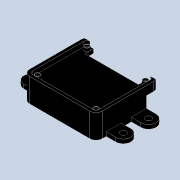
# Autodesk Inventor part: Pi GPIO Mount
Saved by Autodesk Inventor 2022 (Build 260153000, 153)
## iProperties
Created: 2022-01-08
Part Number: Pi GPIO Mount
Material: Generic
Document SubType Name: Modeling
Designer: Coy
Density: 1 g/cm^3
Appearance: Anodized - Black
Author: Coy
Autodesk Inventor part; units mm, degrees
ref_plane "YZ Plane" through (0, 0, 0) normal (1, 0, 0) x (0, 1, 0)
ref_plane "XZ Plane" through (0, 0, 0) normal (0, 1, 0) x (-1, 0, 0)
ref_plane "XY Plane" through (0, 0, 0) normal (0, 0, 1) x (1, 0, 0)
sketch "Sketch1" plane through (0, 0, 0) normal (0, 1, 0) x (-1, 0, 0)
  line L0 (2.5, 0) -> (62.5, 0)
  line L1 (65, 37.5) -> (65, 53.5)
  line L2 (62.5, 56) -> (2.5, 56)
  line L3 (0, 53.5) -> (0, 2.5)
  line L4 (64.5, 37) -> (63, 37)
  line L5 (62.5, 36.5) -> (62.5, 19.5)
  line L6 (63, 19) -> (64.5, 19)
  line L7 (62.5, 37) -> (62.5, 56) construction
  line L8 (62.5, 19) -> (62.5, 0) construction
  arc A0 (65, 53.5) -> (62.5, 56) centre (62.5, 53.5) ccw
  arc A1 (62.5, 0) -> (65, 2.5) centre (62.5, 2.5) ccw
  arc A2 (0, 2.5) -> (2.5, 0) centre (2.5, 2.5) ccw
  arc A3 (2.5, 56) -> (0, 53.5) centre (2.5, 53.5) ccw
  arc A4 (64.5, 37) -> (65, 37.5) centre (64.5, 37.5) ccw
  arc A5 (63, 37) -> (62.5, 36.5) centre (63, 36.5) ccw
  arc A6 (62.5, 19.5) -> (63, 19) centre (63, 19.5) ccw
  line L9 (65, 18.5) -> (65, 2.5)
  arc A7 (65, 18.5) -> (64.5, 19) centre (64.5, 18.5) ccw
  line L10 (59, 0) -> (6, 0)
  line L11 (6, -0.5) -> (6, 8)
  line L12 (6, 8) -> (59, 8)
  line L13 (59, 8) -> (59, -0.5)
  line L14 (59, 8) -> (65, 8) construction
  line L15 (6, 8) -> (0, 8) construction
  line L16 (65.5, 53.5) -> (65.5, 37.5)
  arc A8 (64.5, 36.5) -> (65.5, 37.5) centre (64.5, 37.5) ccw
  line L17 (64.5, 36.5) -> (63, 36.5)
  line L18 (63, 36.5) -> (63, 19.5)
  line L19 (63, 19.5) -> (64.5, 19.5)
  arc A9 (65.5, 18.5) -> (64.5, 19.5) centre (64.5, 18.5) ccw
  line L20 (65.5, 18.5) -> (65.5, 2.5)
  arc A10 (62.5, -0.5) -> (65.5, 2.5) centre (62.5, 2.5) ccw
  line L21 (62.5, -0.5) -> (2.5, -0.5)
  arc A11 (-0.5, 2.5) -> (2.5, -0.5) centre (2.5, 2.5) ccw
  line L22 (-0.5, 2.5) -> (-0.5, 53.5)
  arc A12 (2.5, 56.5) -> (-0.5, 53.5) centre (2.5, 53.5) ccw
  line L23 (2.5, 56.5) -> (62.5, 56.5)
  arc A13 (65.5, 53.5) -> (62.5, 56.5) centre (62.5, 53.5) ccw
  line L24 (65.5, 37.5) -> (65.5, 18.5)
  point P0 (0, 0)
  point P1 (65, 56)
  point P2 (65, 0)
  point P3 (0, 56)
  point P4 (65, 19)
  dimension "d0" = 65
  dimension "d1" = 56
  dimension "d2" = 2.5
  dimension "d3" = 18
  dimension "d4" = 2.5
  dimension "d5" = 0.5
  dimension "d6" = 0.5
  dimension "d7" = 53
  dimension "d9" = 0.5
  dimension "d10" = 8
  constraints: 50 end point, 28 point on circle, 27 point on line, 17 tangent, 14 centre point, 8 parallel, 7 perpendicular, 5 equal radius, 3 horizontal, 2 collinear, 1 vertical, 13 other
  measures "d0" distance of point (0, 56) point (65, 56)
  measures "d1" distance of point (65, 56) point (65, 0)
  measures "d2" distance of point (65, 19) L8.start
  measures "d3" distance of L8.start L7.start
  measures "d4" radius of A0
  measures "d5" radius of A4
  measures "d6" radius of A7
  measures "d7" distance of L11.end L12.end
  measures "d9" distance between parallel lines of L1 L16
  measures "d10" distance between parallel lines of L0 L12
extrude "Extrusion1" add sketch "Sketch1" along normal blind 4 contours A2 L3 A3 L2 A0 L1 A4 L4 A5 L5 A6 L6 A7 L9 A1 L0 L13 L12 L11 | L0 L11 L21 A11 L22 A12 L23 A13 L16 A8 L17 L18 L19 A9 L20 A10 L13 A1 L9 A7 L6 A6 L5 A5 L4 A4 L1 A0 L2 A3 L3 A2 | A9 L19 L18 L17 A8 L24
sketch "Sketch2" plane through (0, 4, 0) normal (0, 1, 0) x (1, 0, 0)
  line L0 (-61.5, -52.5) -> (-3.5, -52.5) construction
  line L1 (-3.5, -52.5) -> (-3.5, -3.5) construction
  line L2 (-3.5, -3.5) -> (-61.5, -3.5) construction
  line L3 (-61.5, -3.5) -> (-61.5, -52.5) construction
  line L4 (-65.5, -2.5) -> (-65.5, -53.5) construction
  arc A0 (-65.5, -53.5) -> (-62.5, -56.5) centre (-62.5, -53.5) ccw construction
  line L5 (-62.5, -56.5) -> (-2.5, -56.5) construction
  arc A1 (-2.5, -56.5) -> (0.5, -53.5) centre (-2.5, -53.5) ccw construction
  line L6 (0.5, -53.5) -> (0.5, -2.5) construction
  arc A2 (0.5, -2.5) -> (-2.5, 0.5) centre (-2.5, -2.5) ccw construction
  line L7 (-2.5, 0.5) -> (-6, 0.5) construction
  line L8 (-6, 0.5) -> (-6, -8) construction
  line L9 (-6, -8) -> (-59, -8) construction
  line L10 (-59, -8) -> (-59, 0.5) construction
  line L11 (-59, 0.5) -> (-62.5, 0.5) construction
  arc A3 (-62.5, 0.5) -> (-65.5, -2.5) centre (-62.5, -2.5) ccw construction
  line L12 (-61.5, -28) -> (-65.5, -28) construction
  line L13 (-65.5, -2.5) -> (-65.5, -53.5) construction
  line L14 (-32.5, -52.5) -> (-32.5, -56.5) construction
  line L15 (-62.5, -56.5) -> (-2.5, -56.5) construction
  line L16 (-3.5, -26.1525) -> (0.5, -26.1525) construction
  line L17 (0.5, -53.5) -> (0.5, -2.5) construction
  line L18 (-5.4848, -3.5) -> (-5.4848, 0.5) construction
  line L19 (-2.5, 0.5) -> (-6, 0.5) construction
  circle A4 centre (-61.5, -52.5) radius 1.1
  circle A5 centre (-61.5, -3.5) radius 1.1
  circle A6 centre (-3.5, -52.5) radius 1.1
  circle A7 centre (-3.5, -3.5) radius 1.1
  circle A8 centre (-61.5, -52.5) radius 2.5
  circle A9 centre (-61.5, -3.5) radius 2.5
  circle A10 centre (-3.5, -3.5) radius 2.5
  circle A11 centre (-3.5, -52.5) radius 2.5
  point P0 (0, 0)
  dimension "d13" = 58
  dimension "d14" = 49
  dimension "d15" = 2.2
  dimension "d16" = 2.2
  dimension "d17" = 2.2
  dimension "d18" = 2.2
  dimension "d19" = 5
  dimension "d20" = 5
  dimension "d21" = 5
  dimension "d22" = 5
  constraints: 16 end point, 8 centre point, 8 coincident, 5 perpendicular, 4 midpoint, 4 parallel, 4 point on line, 1 horizontal
  measures "d13" distance of L2.end L1.end
  measures "d14" distance of L1.end L0.end
  measures "d15" diameter of A4
  measures "d16" diameter of A5
  measures "d17" diameter of A6
  measures "d18" diameter of A7
  measures "d19" diameter of A8
  measures "d20" diameter of A11
  measures "d21" diameter of A9
  measures "d22" diameter of A10
extrude "Extrusion2" add sketch "Sketch2" along normal blind 3
sketch "Sketch3" plane through (-3.5, 4, 3.5) normal (0, 1, 0) x (1, 0, 0)
  circle A0 centre (0, 0) radius 1.1 projected
  circle A1 centre (0, -49) radius 1.1 projected
  circle A2 centre (-58, -49) radius 1.1 projected
  circle A3 centre (-58, 0) radius 1.1 projected
  point P0 (3.5, 3.5)
extrude "Extrusion3" cut sketch "Sketch3" against normal blind 4
sketch "Sketch4" plane through (0, 0, 0) normal (0, -1, 0) x (1, 0, 0)
  circle A0 centre (-61.5, 52.5) radius 1.1 projected
  circle A1 centre (-3.5, 52.5) radius 1.1 projected
  circle A2 centre (-61.5, 3.5) radius 1.1 projected
  circle A3 centre (-3.5, 3.5) radius 1.1 projected
  line L0 (-65.5, 2.5) -> (-65.5, 53.5) projected
  arc A4 (-65.5, 2.5) -> (-62.5, -0.5) centre (-62.5, 2.5) ccw projected
  line L1 (-59, -0.5) -> (-62.5, -0.5) projected
  line L2 (-59, 8) -> (-59, -0.5) projected
  line L3 (-6, 8) -> (-59, 8) projected
  line L4 (-6, -0.5) -> (-6, 8) projected
  line L5 (-2.5, -0.5) -> (-6, -0.5) projected
  arc A5 (-2.5, -0.5) -> (0.5, 2.5) centre (-2.5, 2.5) ccw projected
  line L6 (0.5, 53.5) -> (0.5, 2.5) projected
  arc A6 (0.5, 53.5) -> (-2.5, 56.5) centre (-2.5, 53.5) ccw projected
  line L7 (-62.5, 56.5) -> (-2.5, 56.5) projected
  arc A7 (-62.5, 56.5) -> (-65.5, 53.5) centre (-62.5, 53.5) ccw projected
  line L8 (-68.5, 53.5) -> (-68.5, 2.5)
  arc A8 (-68.5, 2.5) -> (-62.5, -3.5) centre (-62.5, 2.5) ccw
  line L9 (-62.5, -3.5) -> (-56, -3.5)
  line L10 (-56, -3.5) -> (-56, 5)
  line L11 (-56, 5) -> (-9, 5)
  line L12 (-9, 5) -> (-9, -3.5)
  line L13 (-9, -3.5) -> (-2.5, -3.5)
  arc A9 (-2.5, -3.5) -> (3.5, 2.5) centre (-2.5, 2.5) ccw
  line L14 (3.5, 2.5) -> (3.5, 53.5)
  arc A10 (3.5, 53.5) -> (-2.5, 59.5) centre (-2.5, 53.5) ccw
  line L15 (-2.5, 59.5) -> (-62.5, 59.5)
  arc A11 (-62.5, 59.5) -> (-68.5, 53.5) centre (-62.5, 53.5) ccw
  line L16 (-67.6962, -0.5) -> (2.6962, -0.5)
  point P0 (0, 0)
  point P1 (-62.5, -0.5)
  dimension "d27" = 3
  constraints: 18 end point, 10 point on circle, 4 centre point, 1 horizontal, 11 other
  measures "d27" distance between parallel lines of L0 L8
extrude "Extrusion4" add sketch "Sketch4" against normal blind 8.65 contours A4 L16 A8 L8 A11 L15 A10 L14 A9 A5 L6 A6 L7 A7 L0
sketch "Sketch5" plane through (0, 0, 0) normal (0, -1, 0) x (1, 0, 0)
  circle A0 centre (-61.5, 52.5) radius 1.1 projected
  circle A1 centre (-3.5, 52.5) radius 1.1 projected
  circle A2 centre (-61.5, 3.5) radius 1.1 projected
  circle A3 centre (-3.5, 3.5) radius 1.1 projected
  line L0 (-6, -0.5) -> (2.6962, -0.5) projected
  arc A4 (2.6962, -0.5) -> (3.5, 2.5) centre (-2.5, 2.5) ccw projected
  line L1 (3.5, 2.5) -> (3.5, 53.5) projected
  arc A5 (3.5, 53.5) -> (-2.5, 59.5) centre (-2.5, 53.5) ccw projected
  line L2 (-2.5, 59.5) -> (-62.5, 59.5) projected
  arc A6 (-62.5, 59.5) -> (-68.5, 53.5) centre (-62.5, 53.5) ccw projected
  line L3 (-68.5, 53.5) -> (-68.5, 2.5) projected
  arc A7 (-68.5, 2.5) -> (-67.6962, -0.5) centre (-62.5, 2.5) ccw projected
  line L4 (-59, -0.5) -> (-67.6962, -0.5) projected
  line L5 (-59, 8) -> (-59, -0.5) projected
  line L6 (-6, 8) -> (-59, 8) projected
  line L7 (-6, -0.5) -> (-6, 8) projected
  line L8 (-68.5, 53.5) -> (-68.5, 2.5) projected
  line L9 (-68.5, 9.5) -> (3.5, 9.5)
  line L10 (3.5, 53.5) -> (3.5, 2.5) projected
  point P0 (0, 0)
  point P1 (3.5, 9.5)
  dimension "d30" = 10
  constraints: 2 end point, 2 point on line, 1 perpendicular
  measures "d30" distance between parallel lines of L4 L9
extrude "Extrusion5" add sketch "Sketch5" along normal blind 15 contours L9 L3 A6 L2 A5 L1
sketch "Sketch6" plane through (0, -15, 0) normal (0, -1, 0) x (1, 0, 0)
  line L0 (-82.5, -4.1741) -> (-82.5, 71.2939) construction
  line L1 (-62.5, 59.5) -> (-2.5, 59.5) construction
  line L2 (-82.5, 17) -> (-68.5, 17) construction
  line L3 (-68.5, 53.5) -> (-68.5, 9.5) construction
  line L4 (-82.5, 42) -> (-68.5, 42) construction
  line L5 (-75.5, 17) -> (-75.5, 42) construction
  line L6 (-6, -0.5) -> (2.6962, -0.5) construction
  circle A0 centre (-78.011, 17) radius 3
  arc A1 (-75.5, 24.0672) -> (-78.011, 9.5) centre (-78.011, 17) ccw
  line L7 (-68.5, 9.5) -> (-78.011, 9.5)
  line L8 (-68.5, 9.5) -> (3.5, 9.5) projected
  line L9 (-68.5, 24.5) -> (-78.011, 24.5)
  line L10 (-75.5, 29.5) -> (-82.5, 29.5) construction
  circle A2 centre (-78.011, 42) radius 3
  arc A3 (-78.011, 49.5) -> (-75.5, 34.9328) centre (-78.011, 42) ccw
  line L11 (-68.5, 49.5) -> (-78.011, 49.5)
  line L12 (-68.5, 34.5) -> (-78.011, 34.5)
  line L13 (-32.5, 59.5) -> (-32.5, 87.6423) construction
  circle A4 centre (13.011, 17) radius 3
  arc A5 (13.011, 9.5) -> (13.011, 24.5) centre (13.011, 17) ccw
  line L14 (3.5, 9.5) -> (13.011, 9.5)
  line L15 (3.5, 24.5) -> (13.011, 24.5)
  line L16 (3.5, 34.5) -> (13.011, 34.5)
  arc A6 (13.011, 34.5) -> (13.011, 49.5) centre (13.011, 42) ccw
  circle A7 centre (13.011, 42) radius 3
  line L17 (3.5, 49.5) -> (13.011, 49.5)
  line L18 (3.5, 53.5) -> (3.5, 2.5) projected
  line L19 (-68.5, 2.5) -> (-68.5, 53.5) projected
  point P0 (0, 0)
  point P1 (17.5, 17)
  point P2 (10.5, 17)
  point P3 (10.5, 42)
  dimension "d33" = 50
  dimension "d34" = 60
  dimension "d35" = 30
  dimension "d36" = 25
  dimension "d37" = 6
  constraints: 28 end point, 18 symmetric about line, 10 point on circle, 9 point on line, 8 centre point, 4 midpoint, 3 perpendicular, 2 horizontal, 2 tangent, 2 vertical, 1 collinear, 7 other
  measures "d33" distance from line of L0 L13.start
  measures "d34" distance between parallel lines of L1 L6
  measures "d35" distance from line of L1 L10.start
  measures "d36" distance of L5.start L5.end
  measures "d37" diameter of A0
extrude "Extrusion6" add sketch "Sketch6" against normal blind 4
fillet "Fillet1" radius 1 4 edges at (-4.6, 7, 52.5) (-62.6, 7, 52.5) (-4.6, 7, 3.5) (-62.6, 7, 3.5)
equation "\"d5\" = d6"
equation "\"d16\" = d15"
equation "\"d17\" = d15"
equation "\"d18\" = d15"
equation "\"d20\" = d19"
equation "\"d21\" = d19"
equation "\"d22\" = d19"
equation "\"d35\" = 0.5 * d34"
body "Solid1"
